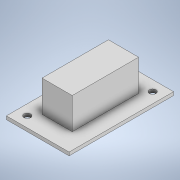
# Autodesk Inventor part: relais
Saved by Autodesk Inventor 2021 (Build 250183000, 183)
## iProperties
Created: 2021-11-10
Part Number: relais
Material: Generisch
Document SubType Name: Modeling
Designer: Simon
Density: 1 g/cm^3
Appearance: Vorgabe
Author: Simon
Autodesk Inventor part; units mm, degrees
ref_plane "YZ Plane" through (0, 0, 0) normal (1, 0, 0) x (0, 1, 0)
ref_plane "XZ Plane" through (0, 0, 0) normal (0, 1, 0) x (-1, 0, 0)
ref_plane "XY Plane" through (0, 0, 0) normal (0, 0, 1) x (1, 0, 0)
sketch "Skizze1" plane through (0, 0, 0) normal (0, 1, 0) x (-1, 0, 0)
  line L0 (15, 25) -> (-15, 25)
  line L1 (-15, 25) -> (-15, -25)
  line L2 (-15, -25) -> (15, -25)
  line L3 (15, -25) -> (15, 25)
  point P0 (0, 0)
  point P1 (15, 0)
  point P2 (0, 25)
  dimension "d0" = 30
  dimension "d1" = 50
  constraints: 8 end point, 2 midpoint, 2 parallel, 1 horizontal, 1 horizontal alignment, 1 perpendicular, 1 vertical alignment
  measures "d0" distance between parallel lines of L1 L3
  measures "d1" distance between parallel lines of L0 L2
extrude "Extrusion1" add sketch "Skizze1" along normal blind 1.6
sketch "Skizze3" plane through (0, 0, 0) normal (0, -1, 0) x (1, 0, 0)
  line L0 (10, 20) -> (-10, 20) construction
  line L1 (-10, 20) -> (-10, -20) construction
  line L2 (-10, -20) -> (10, -20) construction
  line L3 (10, -20) -> (10, 20) construction
  point P0 (0, 0)
  point P1 (10, 0)
  point P2 (0, 20)
  dimension "d6" = 20
  dimension "d7" = 40
  constraints: 8 end point, 3 coincident, 2 midpoint, 2 parallel, 1 horizontal, 1 horizontal alignment, 1 perpendicular, 1 vertical alignment
  measures "d6" distance between parallel lines of L1 L3
  measures "d7" distance between parallel lines of L2 L0
hole "Bohrung1" at (10, 0, 20) at (-10, 0, 20) at (10, 0, -20) direction (0, 1, 0) diameter 3.2 depth 1.6
sketch "Skizze2" plane through (0, 1.6, 0) normal (0, 1, 0) x (1, 0, 0)
  line L0 (-7.338, -15.9212) -> (7.1156, -15.9212)
  line L1 (7.1156, -15.9212) -> (7.1156, 15.8322)
  line L2 (7.1156, 15.8322) -> (-7.338, 15.8322)
  line L3 (-7.338, 15.8322) -> (-7.338, -15.9212)
  point P0 (0, 0)
  constraints: 8 end point, 2 parallel, 1 horizontal, 1 perpendicular
extrude "Extrusion2" add sketch "Skizze2" along normal blind 15
sketch "Skizze4" plane through (0, 0, 0) normal (0, -1, 0) x (1, 0, 0)
  line L0 (10.2328, 16.5217) -> (-10.2861, 16.5217)
  line L1 (-10.2861, 16.5217) -> (-10.2861, -14.3898)
  line L2 (-10.2861, -14.3898) -> (10.2328, -14.3898)
  line L3 (10.2328, -14.3898) -> (10.2328, 16.5217)
  point P0 (7.1156, 15.9212)
  point P1 (-7.338, -15.8322)
  constraints: 8 end point, 2 parallel, 1 horizontal, 1 perpendicular
extrude "Extrusion3" add sketch "Skizze4" along normal blind 2
